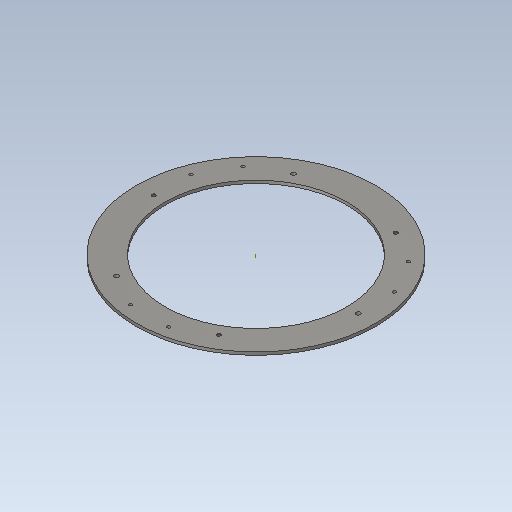
# Autodesk Inventor part: RingPrimaryMirror
Saved by Autodesk Inventor 2020 (Build 240168000, 168)
## iProperties
Created: 2019-04-25
Part Number: RingPrimaryMirror
Material: Stal nierdzewna
Document SubType Name: Modeling
Designer: barto
Density: 8 g/cm^3
Appearance: Częściowo polerowana
Author: barto
Autodesk Inventor part; units mm, degrees
ref_plane "YZ Plane" through (0, 0, 0) normal (1, 0, 0) x (0, 1, 0)
ref_plane "XZ Plane" through (0, 0, 0) normal (0, 1, 0) x (-1, 0, 0)
ref_plane "XY Plane" through (0, 0, 0) normal (0, 0, 1) x (1, 0, 0)
sketch "Szkic3" plane through (0, 0, 0) normal (0, 1, 0) x (-1, 0, 0)
  circle A0 centre (0, 0) radius 125
  circle A1 centre (0, 0) radius 95
  dimension "d14" = 190
  constraints: 2 centre point, 2 coincident
  measures "d14" diameter of A1
extrude "Wyciągnięcie proste3" add sketch "Szkic3" along normal blind 3
sketch "Szkic4" plane through (0, 0, 0) normal (0, -1, 0) x (1, 0, 0)
  circle A0 centre (0, 0) radius 113
  line L0 (0, 0) -> (0, 141.0619)
  point P0 (20, 111.216)
  point P1 (-20, 111.216)
  point P2 (-106.3159, -38.2875)
  point P3 (-86.3159, -72.9285)
  point P4 (86.3159, -72.9285)
  point P5 (106.3159, -38.2875)
  dimension "d23" = 226
  dimension "d24" = 20
  dimension "d25" = 20
  dimension "d96" = 360
  constraints: 2 end point, 2 point on circle, 1 centre point, 1 coincident, 1 vertical, 7 other
  measures "d23" diameter of A0
  measures "d24" distance from line of L0 A0.start
  measures "d25" distance from line of L0 A0.end
sketch "Szkic7" plane through (0, 0, 0) normal (0, -1, 0) x (1, 0, 0)
  circle A0 centre (0, 0) radius 106.9
  point P0 (106.9, 0)
  point P1 (-53.45, 92.5781)
  point P2 (-53.45, -92.5781)
  dimension "d69" = 213.8
  dimension "d72" = 360
  constraints: 1 coincident, 1 horizontal alignment, 6 other
hole "Otwór2" at (106.9, 0, 0) at (-53.45, 0, 92.5781) at (-53.45, 0, -92.5781) direction (0, 1, 0) diameter 4.5 end through all clearance for "Śruba ze łbem stożkowym ISO 2009/7046" size "M4" standard "ISO"
sketch "Szkic9" plane through (0, 0, 0) normal (0, -1, 0) x (1, 0, 0)
  point P0 (0, 0)
  point P1 (53.45, -92.5781)
  point P2 (53.45, 92.5781)
  point P3 (-106.9, 0)
  dimension "d85" = 360
  constraints: 4 other
hole "Otwór3" at (53.45, 0, -92.5781) at (53.45, 0, 92.5781) at (-106.9, 0, 0) direction (0, 1, 0) diameter 3.242 end through all thread size "M4x0.7" class "6H" standard "ISO Metric profile"
hole "Otwór4" at (20, 0, 111.216) at (-20, 0, 111.216) at (-106.3159, 0, -38.2875) at (-86.3159, 0, -72.9285) at (86.3159, 0, -72.9285) at (106.3159, 0, -38.2875) direction (0, 1, 0) diameter 3.4 end through all clearance for "Śruba ze łbem stożkowym ISO 2009/7046" size "M3" standard "ISO"
chamfer "Faza1" distance 0.4 angle 45 9 edges at (86.3159, 0, -71.2285) (106.3159, 0, -36.5875) (-86.3159, 0, -71.2285) (-106.3159, 0, -36.5875) (20, 0, 112.916) (-20, 0, 112.916) (53.45, 3, -90.9571) (-106.9, 3, 1.621) (53.45, 3, 94.1991)
